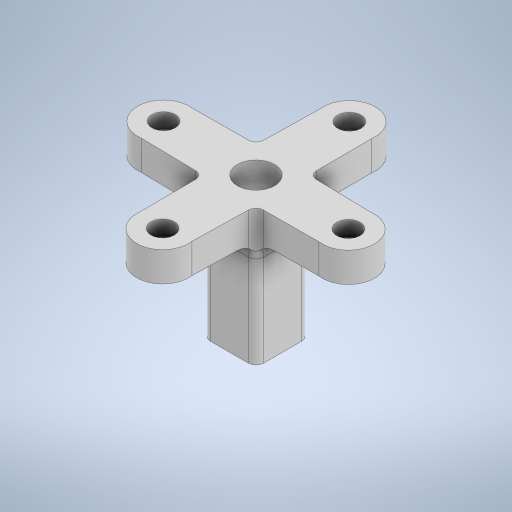
# Autodesk Inventor part: franka_mount
Saved by Autodesk Inventor 2023.1 (Build 271208000, 208)
## iProperties
Created: 2022-08-07
Part Number: franka_mount
Material: Generic
Document SubType Name: Modeling
Designer: fraaw
Density: 1 g/cm^3
Appearance: Default
Author: fraaw
## iProperties of the stored document franka_mount_3DPrint.ipt
Created: 2022-08-07
Part Number: franka_mount_3DPrint
Material: Generic
Document SubType Name: Modeling
Designer: fraaw
Density: 1 g/cm^3
Appearance: Default
Author: fraaw
Autodesk Inventor part; units mm, degrees
ref_plane "YZ Plane" through (0, 0, 0) normal (1, 0, 0) x (0, 1, 0)
ref_plane "XZ Plane" through (0, 0, 0) normal (0, 1, 0) x (-1, 0, 0)
ref_plane "XY Plane" through (0, 0, 0) normal (0, 0, 1) x (1, 0, 0)
sketch "Sketch1" plane through (0, 0, 0) normal (0, 1, 0) x (-1, 0, 0)
  line L0 (5.15, 5.15) -> (-5.15, 5.15)
  line L1 (-5.15, 5.15) -> (-5.15, -5.15)
  line L2 (-5.15, -5.15) -> (5.15, -5.15)
  line L3 (5.15, -5.15) -> (5.15, 5.15)
  line L4 (5.15, 5.15) -> (-5.15, -5.15) construction
  line L5 (-5.15, 5.15) -> (5.15, -5.15) construction
  line L6 (-7.15, 7.15) -> (7.15, 7.15)
  line L7 (7.15, 7.15) -> (7.15, -7.15)
  line L8 (7.15, -7.15) -> (-7.15, -7.15)
  line L9 (-7.15, -7.15) -> (-7.15, 7.15)
  point P0 (0, 0)
  dimension "d0" = 10.3
  dimension "d1" = 10.3
  dimension "d4" = 2
  constraints: 20 end point, 4 parallel, 2 midpoint, 2 perpendicular, 1 horizontal, 3 other
  measures "d0" distance of L1.end L2.end
  measures "d1" distance of L2.end L0.start
  measures "d4" distance between parallel lines of L0 L6
extrude "Extrusion1" add sketch "Sketch1" along normal blind 29.7
sketch "Sketch2" plane through (0, 29.7, 0) normal (0, 1, 0) x (1, 0, 0)
  circle A0 centre (0, 0) radius 25 construction
  circle A1 centre (0.126, 24.9997) radius 3.125
  arc A2 (7.0521, 23.9848) -> (-6.8099, 24.0546) centre (0.126, 24.9997) ccw
  line L0 (-7.15, 7.15) -> (-7.15, -7.15) projected
  line L1 (7.15, -7.15) -> (7.15, 7.15) projected
  line L2 (7.15, 7.15) -> (-7.15, 7.15) construction
  line L3 (-6.8099, 24.0546) -> (-7.15, 7.15)
  line L4 (7.0521, 23.9848) -> (7.15, 7.15)
  circle A3 centre (-24.9997, 0.126) radius 3.125
  arc A4 (-23.9848, 7.0521) -> (-24.0546, -6.8099) centre (-24.9997, 0.126) ccw
  line L5 (-23.9848, 7.0521) -> (-7.15, 7.15)
  line L6 (-24.0546, -6.8099) -> (-7.15, -7.15)
  circle A5 centre (-0.126, -24.9997) radius 3.125
  arc A6 (-7.0521, -23.9848) -> (6.8099, -24.0546) centre (-0.126, -24.9997) ccw
  line L7 (-7.0521, -23.9848) -> (-7.15, -7.15)
  line L8 (6.8099, -24.0546) -> (7.15, -7.15)
  circle A7 centre (24.9997, -0.126) radius 3.125
  arc A8 (23.9848, -7.0521) -> (24.0546, 6.8099) centre (24.9997, -0.126) ccw
  line L9 (23.9848, -7.0521) -> (7.15, -7.15)
  line L10 (24.0546, 6.8099) -> (7.15, 7.15)
  point P0 (7.15, 7.15)
  point P1 (-7.15, 7.15)
  point P2 (-7.15, -7.15)
  point P3 (7.15, -7.15)
  dimension "d5" = 50
  dimension "d6" = 6.25
  dimension "d10" = 360
  dimension "d28" = 7
  constraints: 16 end point, 11 point on circle, 9 centre point, 1 coincident, 37 other
  measures "d5" diameter of A0
  measures "d6" diameter of A1
  measures "d28" radius of A2
extrude "Extrusion2" add sketch "Sketch2" along normal blind 8
sketch "Sketch3" plane through (0, 29.7, 0) normal (0, -1, 0) x (1, 0, 0)
  circle A0 centre (24.9997, 0.126) radius 3.125 projected
  circle A1 centre (24.9997, 0.126) radius 5.1
  circle A2 centre (-0.126, 24.9997) radius 5.1
  circle A3 centre (-24.9997, -0.126) radius 5.1
  circle A4 centre (0.126, -24.9997) radius 5.1
  point P0 (0, 0)
  dimension "d14" = 10.2
  dimension "d17" = 360
  constraints: 4 centre point, 1 coincident, 9 other
  measures "d14" diameter of A1
extrude "Extrusion3" cut sketch "Sketch3" against normal blind 4
sketch "Sketch4" plane through (0, 29.7, 0) normal (0, -1, 0) x (1, 0, 0)
  point P0 (0, 0)
  point P1 (0, 0)
  constraints: 1 coincident
hole "Hole1" at (0, 29.7, 0) direction (0, 1, 0) diameter 10 end through all
fillet "Fillet1" radius 5 4 edges at (0, 29.7, 7.15) (7.15, 29.7, 0) (-7.15, 29.7, 0) (0, 29.7, -7.15)
fillet "Fillet2" radius 2 4 edges at (7.15, 31.2, 7.15) (7.15, 31.2, -7.15) (-7.15, 31.2, -7.15) (-7.15, 31.2, 7.15)
fillet "Fillet3" radius 2 8 edges at (7.2921, 25.8836, 7.2921) (7.15, 12.35, 7.15) (-7.2921, 25.8836, 7.2921) (-7.15, 12.35, 7.15) (-7.2921, 25.8836, -7.2921) (-7.15, 12.35, -7.15) (7.2921, 25.8836, -7.2921) (7.15, 12.35, -7.15)
equation "\"d1\" = d0"
body "Solid1"
